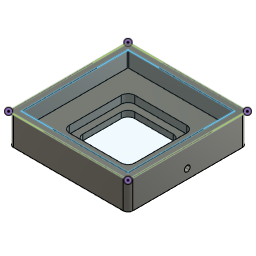
Load cell V4 55 2mm (Autodesk Fusion 360 design; units mm, degrees)
Autodesk Fusion 360 part; units mm, degrees
sketch "Sketch2" plane through (0, 0, 0) normal (0, 1, 0) x (1, 0, 0)
  line L0 (-31, 31) -> (31, 31)
  line L1 (31, 31) -> (31, -31)
  line L2 (31, -31) -> (-31, -31)
  line L3 (-31, -31) -> (-31, 31)
  constraint horizontal L0
  constraint vertical L1
  constraint horizontal L2
  constraint vertical L3
extrude "Extrude1" add sketch "Sketch2" along normal blind 15 makes body 1
ref_plane "WorkPlane1" through (0, 3, 0) normal (0, -1, 0) x (-1, 0, 0)
split "Split1" by plane through (0, 3, 0) normal (0, -1, 0) bodies 1 makes body 2 at (-10.3333, 0, -10.3333)
ref_plane "WorkPlane2" through (0, 7, 0) normal (0, -1, 0) x (-1, 0, 0)
split "Split2" by plane through (0, 7, 0) normal (0, -1, 0) bodies 1 makes body 3 at (-10.3333, 3, 10.3333)
sketch "Sketch3" plane through (0, 15, 0) normal (0, 1, 0) x (-1, 0, 0)
  line L0 (31, 31) -> (-31, 31)
  line L1 (-31, 31) -> (-31, -31)
  line L2 (-31, -31) -> (31, -31)
  line L3 (31, -31) -> (31, 31)
  line L4 (27.6, -27.6) -> (-27.6, -27.6)
  line L5 (-27.6, -27.6) -> (-27.6, 27.6)
  line L6 (-27.6, 27.6) -> (27.6, 27.6)
  line L7 (27.6, 27.6) -> (27.6, -27.6)
  line L8 (31, 31) -> (-31, 31)
  line L9 (-31, 31) -> (-31, -31)
  line L10 (-31, -31) -> (31, -31)
  line L11 (31, -31) -> (31, 31)
  constraint horizontal L4
  constraint vertical L5
  constraint horizontal L6
  constraint vertical L7
extrude "Extrude2" cut sketch "Sketch3" against normal blind 8 contours L4 L5 L6 L7 bodies 1
sketch "Sketch4" plane through (0, 7, 0) normal (0, 1, 0) x (-1, 0, 0)
  line L0 (31, 31) -> (-31, 31)
  line L1 (-31, 31) -> (-31, -31)
  line L2 (-31, -31) -> (31, -31)
  line L3 (31, -31) -> (31, 31)
  line L4 (17, -17) -> (-17, -17)
  line L5 (-17, -17) -> (-17, 17)
  line L6 (-17, 17) -> (17, 17)
  line L7 (17, 17) -> (17, -17)
  constraint horizontal L4
  constraint vertical L5
  constraint horizontal L6
  constraint vertical L7
extrude "Extrude3" cut sketch "Sketch4" against normal blind 4 contours L4 L5 L6 L7 bodies 3
fillet "Fillet1" radius 3.5 4 edges at (17, 5, -17) (-17, 5, 17) (-17, 5, -17) (17, 5, 17) on bodies 3
sketch "Sketch6" plane through (0, 3, 0) normal (0, 1, 0) x (-1, 0, 0)
  line L0 (31, -31) -> (31, 31)
  line L1 (31, 31) -> (-31, 31)
  line L2 (-31, 31) -> (-31, -31)
  line L3 (-31, -31) -> (31, -31)
  line L4 (13.5, -13.5) -> (-13.5, -13.5)
  line L5 (-13.5, -13.5) -> (-13.5, 13.5)
  line L6 (-13.5, 13.5) -> (13.5, 13.5)
  line L7 (13.5, 13.5) -> (13.5, -13.5)
  constraint horizontal L4
  constraint vertical L5
  constraint horizontal L6
  constraint vertical L7
extrude "Extrude4" cut sketch "Sketch6" against normal blind 6 contours L4 L5 L6 L7 bodies 2
fillet "Fillet2" radius 3.5 4 edges at (-13.5, 1.5, 13.5) (13.5, 1.5, 13.5) (13.5, 1.5, -13.5) (-13.5, 1.5, -13.5) on bodies 2
hole "Hole1" at (17, 4.8556, 0.2033) direction (1, 0, 0) diameter 3 depth 40 tip angle 180 bodies 3
fillet "Fillet3" radius 0.4 4 edges at (27.6, 11, 27.6) (27.6, 11, -27.6) (-27.6, 11, -27.6) (-27.6, 11, 27.6) on bodies 1
combine "Combine1" operation add target body 1 tool bodies 3
combine "Combine2" operation add target body 1 tool bodies 2
fillet "Fillet4" radius 2.5 4 edges at (31, 7.5, -31) (-31, 7.5, -31) (-31, 7.5, 31) (31, 7.5, 31) on bodies 1
split "Split3" by plane through (0, 7, 0) normal (0, -1, 0) bodies 1 makes body 4 at (-3.3333, 0, 25.1667)
combine "Combine3" operation add target body 1 tool bodies 4
split "Split4" by plane through (0, 7, 0) normal (0, -1, 0) bodies 1 makes body 5 at (-3.3333, 0, 25.1667)
combine "Combine4" operation add target body 1 tool bodies 5
split "Split5" by plane through (0, 7, 0) normal (0, -1, 0) bodies 1 makes body 6 at (-3.3333, 0, 25.1667)
combine "Combine5" operation add target body 1 tool bodies 6
